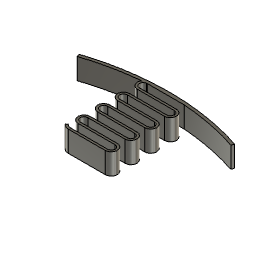
Coupler_Spring (Autodesk Fusion 360 design; units mm, degrees)
Autodesk Fusion 360 part; units mm, degrees
sketch "Spring Sweep Path" plane through (0, 0, 0) normal (0, 0, 1) x (1, 0, 0)
  line L0 (-3.75, 0) -> (3.75, 0)
  line L1 (-3.75, -8) -> (3.75, -8)
  line L2 (-3.75, -6) -> (3.75, -6)
  line L3 (-3.75, -4) -> (3.75, -4)
  line L4 (-3.75, -2) -> (3.75, -2)
  line L5 (-3.75, 2) -> (3.75, 2)
  line L6 (-3.75, 4) -> (3.75, 4)
  line L7 (-3.75, 6) -> (3.75, 6)
  line L8 (-3.75, 8) -> (3.75, 8)
  arc A0 (3.75, -8) -> (3.75, -6) centre (3.75, -7) ccw
  arc A1 (-3.75, -4) -> (-3.75, -6) centre (-3.75, -5) ccw
  arc A2 (3.75, -4) -> (3.75, -2) centre (3.75, -3) ccw
  arc A3 (-3.75, 0) -> (-3.75, -2) centre (-3.75, -1) ccw
  arc A4 (3.75, 0) -> (3.75, 2) centre (3.75, 1) ccw
  arc A5 (-3.75, 4) -> (-3.75, 2) centre (-3.75, 3) ccw
  arc A6 (3.75, 4) -> (3.75, 6) centre (3.75, 5) ccw
  arc A7 (-3.75, 8) -> (-3.75, 6) centre (-3.75, 7) ccw
  arc A8 (-4.75, -7.5) -> (-3.75, -8) centre (-3.75, -6.75) ccw
  line L9 (-4.75, -7.5) -> (4.616, -7.5) construction
  line L10 (-4.75, -5) -> (-4.75, -7.5) construction
  dimension "d1" = 7.5
  dimension "d4" = 0
  dimension "d5" = 2
  dimension "d6" = 0.5
  constraint horizontal L0
  constraint midpoint origin L0
  constraint tangent L1 A0
  constraint tangent L2 A1
  constraint tangent L3 A2
  constraint tangent L4 A3
  constraint tangent L0 A4
  constraint tangent L5 A5
  constraint tangent L6 A6
  constraint tangent L7 A7
  constraint tangent L1 A8
  constraint horizontal L9
  constraint midpoint A1 L10.start
  constraint vertical L10
  constraint coincident A0 L9.end
  measures "d1" distance of L0.start L0.end
  measures "d6" distance of L1 L9
sketch "Spring Sweep Object" plane through (0, 0, 0) normal (1, 0, 0) x (0, 1, 0)
  line L0 (-0.225, 4.25) -> (0.225, 4.25)
  line L1 (0.225, 4.25) -> (0.225, 0)
  line L2 (0.225, 0) -> (-0.225, 0)
  line L3 (-0.225, 0) -> (-0.225, 4.25)
  dimension "d7" = 0.45
  dimension "d8" = 4.25
  constraint horizontal L0
  constraint vertical L1
  constraint horizontal L2
  constraint vertical L3
  constraint midpoint L2 origin
  measures "d7" distance of L0.start L0.end
  measures "d8" distance of L0.start L2.end
sweep "Sweep1" add profiles "Spring Sweep Object" path "Spring Sweep Path" along A8 L1 A0 L2 A1 L3 A2 L4 A3 L0 A4 L5 A5 L6 A6 L7 A7 L8 section 1
sketch "Curved Head" plane through (0, 0, 0) normal (0, 0, 1) x (1, 0, 0)
  line L0 (-3.75, -0.225) -> (3.75, -0.225) construction
  arc A0 (3.75, -0.225) -> (3.75, 2.225) centre (3.75, 1) ccw construction
  line L1 (3.75, 2.225) -> (-3.75, 2.225) construction
  arc A1 (-3.75, 3.775) -> (-3.75, 2.225) centre (-3.75, 3) ccw construction
  line L2 (-3.75, 3.775) -> (3.75, 3.775) construction
  arc A2 (3.75, 3.775) -> (3.75, 6.225) centre (3.75, 5) ccw construction
  line L3 (3.75, 6.225) -> (-3.75, 6.225) construction
  arc A3 (-3.75, 7.775) -> (-3.75, 6.225) centre (-3.75, 7) ccw construction
  line L4 (-3.75, 7.775) -> (3.75, 7.775) construction
  line L5 (3.75, 7.775) -> (3.75, 8.225) construction
  line L6 (3.75, 8.225) -> (-3.75, 8.225) construction
  arc A4 (-3.75, 8.225) -> (-3.75, 5.775) centre (-3.75, 7) ccw construction
  line L7 (-3.75, 5.775) -> (3.75, 5.775) construction
  arc A5 (3.75, 4.225) -> (3.75, 5.775) centre (3.75, 5) ccw construction
  line L8 (3.75, 4.225) -> (-3.75, 4.225) construction
  arc A6 (-3.75, 4.225) -> (-3.75, 1.775) centre (-3.75, 3) ccw construction
  line L9 (-3.75, 1.775) -> (3.75, 1.775) construction
  arc A7 (3.75, 0.225) -> (3.75, 1.775) centre (3.75, 1) ccw construction
  line L10 (3.75, 0.225) -> (-3.75, 0.225) construction
  arc A8 (-3.75, 0.225) -> (-3.75, -2.225) centre (-3.75, -1) ccw construction
  line L11 (-3.75, -2.225) -> (3.75, -2.225) construction
  arc A9 (3.75, -3.775) -> (3.75, -2.225) centre (3.75, -3) ccw construction
  line L12 (3.75, -3.775) -> (-3.75, -3.775) construction
  arc A10 (-3.75, -3.775) -> (-3.75, -6.225) centre (-3.75, -5) ccw construction
  line L13 (-3.75, -6.225) -> (3.75, -6.225) construction
  arc A11 (3.75, -7.775) -> (3.75, -6.225) centre (3.75, -7) ccw construction
  line L14 (3.75, -7.775) -> (-3.75, -7.775) construction
  arc A12 (-4.57, -7.365) -> (-3.75, -7.775) centre (-3.75, -6.75) ccw construction
  line L15 (-4.57, -7.365) -> (-4.93, -7.635) construction
  arc A13 (-4.93, -7.635) -> (-3.75, -8.225) centre (-3.75, -6.75) ccw construction
  line L16 (-3.75, -8.225) -> (3.75, -8.225) construction
  arc A14 (3.75, -8.225) -> (3.75, -5.775) centre (3.75, -7) ccw construction
  line L17 (3.75, -5.775) -> (-3.75, -5.775) construction
  arc A15 (-3.75, -4.225) -> (-3.75, -5.775) centre (-3.75, -5) ccw construction
  line L18 (-3.75, -4.225) -> (3.75, -4.225) construction
  arc A16 (3.75, -4.225) -> (3.75, -1.775) centre (3.75, -3) ccw construction
  line L19 (3.75, -1.775) -> (-3.75, -1.775) construction
  arc A17 (-3.75, -0.225) -> (-3.75, -1.775) centre (-3.75, -1) ccw construction
  arc A18 (15.75, 6) -> (-15.75, 6) centre (0, -42.0401) ccw
  line L20 (0, -42.0401) -> (0, 7.9159) construction
  arc A19 (15.5631, 5.4299) -> (-15.5631, 5.4299) centre (0, -42.0401) ccw
  line L21 (-15.75, 6) -> (-15.5631, 5.4299)
  line L22 (15.5631, 5.4299) -> (15.75, 6)
  line L23 (-15.5631, 5.4299) -> (0, -42.0401) construction
  line L24 (15.5631, 5.4299) -> (0, -42.0401) construction
  line L25 (-3.75, 6.225) -> (3.75, 5.775) construction
  line L26 (-15.75, 6) -> (15.75, 6) construction
  dimension "d16" = 31.5
  dimension "d18" = 0.6
  constraint perpendicular L6 L20
  constraint concentric A18 A19
  constraint coincident A18.centre L20.start
  constraint collinear L21 L23
  constraint collinear L22 L24
  constraint coincident L3.end A3.end
  constraint coincident L7.end A5.end
  constraint midpoint L25 L26
  constraint coincident L4.end A19
  constraint coincident A3.start A19
  constraint midpoint A19 L20.end
  measures "d16" distance of A18.end A18.start
  measures "d18" distance of A18 A19
extrude "Extrude1" add sketch "Curved Head" along normal up to surface (4.25 mm away)
named bodies: "Spring Body"
